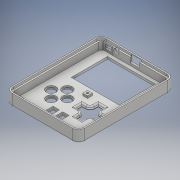
# Autodesk Inventor part: CaseGroboyFront
Saved by Autodesk Inventor 2017 SP1 (Build 210196100, 196)
## iProperties
Created: 2017-08-23
Part Number: CaseGroboyFront
Material: Generic
Document SubType Name: Modeling
Designer: Groguard
Density: 1 g/cm^3
Appearance: Default
Author: Groguard
Autodesk Inventor part; units mm, degrees
ref_plane "YZ Plane" through (0, 0, 0) normal (1, 0, 0) x (0, 1, 0)
ref_plane "XZ Plane" through (0, 0, 0) normal (0, 1, 0) x (-1, 0, 0)
ref_plane "XY Plane" through (0, 0, 0) normal (0, 0, 1) x (1, 0, 0)
sketch "Sketch1" plane through (0, 0, 0) normal (0, 0, 1) x (1, 0, 0)
  line L0 (50, 18.25) -> (50, 11.75)
  arc A0 (50.0508, 18.25) -> (49.9492, 18.25) centre (50, 18.25) ccw
  line L1 (50, 11.75) -> (44, 11.75)
  line L2 (44, 11.75) -> (44, 18.25)
  arc A1 (44.0508, 18.25) -> (43.9492, 18.25) centre (44, 18.25) ccw
  line L3 (44, 18.25) -> (50, 18.25)
  arc A2 (50, 18.1992) -> (50, 18.3008) centre (50, 18.25) ccw
  arc A3 (44, 18.3008) -> (44, 18.1992) centre (44, 18.25) ccw
  line L4 (38, 18.25) -> (38, 11.75)
  arc A4 (38.0508, 18.25) -> (37.9492, 18.25) centre (38, 18.25) ccw
  line L5 (38, 11.75) -> (32, 11.75)
  line L6 (32, 11.75) -> (32, 18.25)
  arc A5 (32.0508, 18.25) -> (31.9492, 18.25) centre (32, 18.25) ccw
  line L7 (32, 18.25) -> (38, 18.25)
  arc A6 (38, 18.1992) -> (38, 18.3008) centre (38, 18.25) ccw
  arc A7 (32, 18.3008) -> (32, 18.1992) centre (32, 18.25) ccw
  line L8 (3.96, 108.28) -> (73.16, 108.28)
  arc A8 (73.16, 108.2482) -> (73.16, 108.3118) centre (73.16, 108.28) ccw
  arc A9 (3.96, 108.3118) -> (3.96, 108.2482) centre (3.96, 108.28) ccw
  line L9 (73.16, 108.28) -> (73.16, 58.28)
  arc A10 (73.1282, 58.28) -> (73.1917, 58.28) centre (73.16, 58.28) ccw
  arc A11 (73.1917, 108.28) -> (73.1282, 108.28) centre (73.16, 108.28) ccw
  line L10 (73.16, 58.28) -> (3.96, 58.28)
  arc A12 (3.96, 58.3118) -> (3.96, 58.2482) centre (3.96, 58.28) ccw
  arc A13 (73.16, 58.2482) -> (73.16, 58.3118) centre (73.16, 58.28) ccw
  line L11 (3.96, 58.28) -> (3.96, 108.28)
  arc A14 (3.9918, 108.28) -> (3.9283, 108.28) centre (3.96, 108.28) ccw
  arc A15 (3.9283, 58.28) -> (3.9918, 58.28) centre (3.96, 58.28) ccw
  line L12 (32, 18.25) -> (38, 18.25)
  line L13 (38, 18.25) -> (38, 11.75)
  line L14 (38, 11.75) -> (32, 11.75)
  line L15 (32, 11.75) -> (32, 18.25)
  line L16 (44, 18.25) -> (50, 18.25)
  line L17 (50, 18.25) -> (50, 11.75)
  line L18 (50, 11.75) -> (44, 11.75)
  line L19 (44, 11.75) -> (44, 18.25)
  arc A16 (83, 106.5858) -> (78.5858, 111) centre (78.5858, 106.5858) ccw
  line L20 (83, 106.5858) -> (83, 3.4142)
  arc A17 (78.5858, -1) -> (83, 3.4142) centre (78.5858, 3.4142) ccw
  line L21 (78.5858, -1) -> (3.4142, -1)
  arc A18 (-1, 3.4142) -> (3.4142, -1) centre (3.4142, 3.4142) ccw
  line L22 (-1, 3.4142) -> (-1, 106.5858)
  arc A19 (3.4142, 111) -> (-1, 106.5858) centre (3.4142, 106.5858) ccw
  line L23 (3.4142, 111) -> (78.5858, 111)
  arc A20 (86, 106.5858) -> (78.5858, 114) centre (78.5858, 106.5858) ccw
  line L24 (86, 106.5858) -> (86, 3.4142)
  arc A21 (78.5858, -4) -> (86, 3.4142) centre (78.5858, 3.4142) ccw
  line L25 (78.5858, -4) -> (3.4142, -4)
  arc A22 (-4, 3.4142) -> (3.4142, -4) centre (3.4142, 3.4142) ccw
  line L26 (-4, 3.4142) -> (-4, 106.5858)
  arc A23 (3.4142, 114) -> (-4, 106.5858) centre (3.4142, 106.5858) ccw
  line L27 (3.4142, 114) -> (78.5858, 114)
  line L28 (50.75, 39.3006) -> (46.75, 39.3006)
  line L29 (46.75, 39.3006) -> (46.75, 32.8006)
  line L30 (46.75, 32.8006) -> (50.75, 32.8006)
  line L31 (56.75, 26.8006) -> (56.75, 22.8006)
  line L32 (56.75, 45.3006) -> (56.75, 49.3006)
  line L33 (56.75, 49.3006) -> (63.25, 49.3006)
  line L34 (63.25, 49.3006) -> (63.25, 45.3006)
  line L35 (69.25, 39.3006) -> (73.25, 39.3006)
  line L36 (73.25, 39.3006) -> (73.25, 32.8006)
  line L37 (73.25, 32.8006) -> (69.25, 32.8006)
  line L38 (63.25, 26.8006) -> (63.25, 22.8006)
  line L39 (63.25, 22.8006) -> (56.75, 22.8006)
  arc A24 (63.25, 45.3006) -> (69.25, 39.3006) centre (69.25, 45.3006) ccw
  arc A25 (50.75, 39.3006) -> (56.75, 45.3006) centre (50.75, 45.3006) ccw
  arc A26 (56.75, 26.8006) -> (50.75, 32.8006) centre (50.75, 26.8006) ccw
  arc A27 (69.25, 32.8006) -> (63.25, 26.8006) centre (69.25, 26.8006) ccw
  circle A28 centre (22, 46) radius 5
  circle A29 centre (32, 36) radius 5
  circle A30 centre (22, 26) radius 5
  circle A31 centre (12, 36) radius 5
  line L40 (11.35, 60.9) -> (11.35, 105.9)
  line L41 (11.35, 105.9) -> (70.65, 105.9)
  line L42 (70.65, 105.9) -> (70.65, 60.9)
  line L43 (70.65, 60.9) -> (11.35, 60.9)
  point P0 (0, 0)
  point P1 (18.75, 39)
  point P2 (18.75, 32.5)
  point P3 (63.25, 39)
  point P4 (63.25, 32.5)
  constraints: 88 end point, 56 point on circle, 32 centre point, 4 parallel, 3 perpendicular, 2 horizontal, 1 point on line
extrude "Face" add sketch "Sketch1" along normal blind 3 contours L3 A0 A2 L0 | L3 L2 A3 A1 | L7 A4 A6 L4 | L7 L6 A7 A5 | L11 A9 A14 L8 | L8 L9 L10 L11 | A11 A8 L9 L8 | L11 L10 A15 A12 | A13 A10 L10 L9 | L20 A17 L21 A18 L22 A19 L23 A16 | L24 A21 L25 A22 L26 A23 L27 A20 | L40 L41 L42 L43
sketch "Sketch12" plane through (0, 0, 3) normal (0, 0, 1) x (1, 0, 0)
  line L0 (78.5858, 114) -> (3.4142, 114) projected
  line L1 (3.4142, 114) -> (78.5858, 114)
  arc A0 (86, 106.5858) -> (78.5858, 114) centre (78.5858, 106.5858) ccw projected
  arc A1 (86, 106.5858) -> (78.5858, 114) centre (78.5858, 106.5858) ccw
  line L2 (86, 3.4142) -> (86, 106.5858) projected
  line L3 (86, 106.5858) -> (86, 3.4142)
  arc A2 (78.5858, -4) -> (78.5858, -4) centre (78.5858, 3.4142) ccw
  line L4 (78.5858, -4) -> (3.4142, -4) projected
  line L5 (3.4142, -4) -> (78.5858, -4) projected
  line L6 (78.5858, -4) -> (3.4142, -4)
  arc A3 (-4, 3.4142) -> (3.4142, -4) centre (3.4142, 3.4142) ccw projected
  arc A4 (-4, 3.4142) -> (3.4142, -4) centre (3.4142, 3.4142) ccw
  line L7 (-4, 3.4142) -> (-4, 106.5858)
  line L8 (-4, 3.4142) -> (-4, 106.5858) projected
  arc A5 (3.4142, 114) -> (-4, 106.5858) centre (3.4142, 106.5858) ccw
  arc A6 (78.5858, -4) -> (86, 3.4142) centre (78.5858, 3.4142) ccw
  line L9 (-1, 106.5858) -> (-1, 3.4142)
  arc A7 (-1, 3.4142) -> (3.4142, -1) centre (3.4142, 3.4142) ccw
  line L10 (3.4142, -1) -> (78.5858, -1)
  arc A8 (78.5858, -1) -> (83, 3.4142) centre (78.5858, 3.4142) ccw
  line L11 (83, 3.4142) -> (83, 106.5858)
  arc A9 (83, 106.5858) -> (78.5858, 111) centre (78.5858, 106.5858) ccw
  line L12 (78.5858, 111) -> (3.4142, 111)
  arc A10 (3.4142, 111) -> (-1, 106.5858) centre (3.4142, 106.5858) ccw
  point P0 (0, 0)
  dimension "d70" = 3
  constraints: 16 end point, 16 point on circle, 8 centre point, 3 collinear, 1 vertical, 1 vertical alignment, 10 other
  measures "d70" radial gap between concentric circles of A5 A10
extrude "Walls" add sketch "Sketch12" along normal blind 12 contours A0 L2 A2 L11 A9 L12 A10 L9 A7 L10 L4 A3 L7 A5 L0 | A2 L10 A8 L11 picked at (75.0084, -1.4191)
sketch "Sketch14" plane through (0, 0, 15) normal (0, 0, 1) x (1, 0, 0)
  line L0 (78.5858, 114) -> (3.4142, 114)
  arc A0 (86, 106.5858) -> (78.5858, 114) centre (78.5858, 106.5858) ccw
  line L1 (86, 3.4142) -> (86, 106.5858)
  line L2 (3.4142, -4) -> (78.5858, -4)
  arc A1 (-4, 3.4142) -> (3.4142, -4) centre (3.4142, 3.4142) ccw
  line L3 (-4, 3.4142) -> (-4, 106.5858)
  arc A2 (3.4142, 114) -> (-4, 106.5858) centre (3.4142, 106.5858) ccw
  arc A3 (78.5858, -4) -> (86, 3.4142) centre (78.5858, 3.4142) ccw
  line L4 (-2.5, 106.5858) -> (-2.5, 3.4142)
  arc A4 (-2.5, 3.4142) -> (3.4142, -2.5) centre (3.4142, 3.4142) ccw
  line L5 (3.4142, -2.5) -> (78.5858, -2.5)
  arc A5 (78.5858, -2.5) -> (84.5, 3.4142) centre (78.5858, 3.4142) ccw
  line L6 (84.5, 3.4142) -> (84.5, 106.5858)
  arc A6 (84.5, 106.5858) -> (78.5858, 112.5) centre (78.5858, 106.5858) ccw
  line L7 (78.5858, 112.5) -> (3.4142, 112.5)
  arc A7 (3.4142, 112.5) -> (-2.5, 106.5858) centre (3.4142, 106.5858) ccw
  line L8 (-1, 106.5858) -> (-1, 3.4142)
  arc A8 (-1, 3.4142) -> (3.4142, -1) centre (3.4142, 3.4142) ccw
  line L9 (3.4142, -1) -> (78.5858, -1)
  arc A9 (78.5858, -1) -> (83, 3.4142) centre (78.5858, 3.4142) ccw
  line L10 (83, 3.4142) -> (83, 106.5858)
  arc A10 (83, 106.5858) -> (78.5858, 111) centre (78.5858, 106.5858) ccw
  line L11 (78.5858, 111) -> (3.4142, 111)
  arc A11 (3.4142, 111) -> (-1, 106.5858) centre (3.4142, 106.5858) ccw
  point P0 (0, 0)
  dimension "d73" = 1.5
  dimension "d74" = 3
  constraints: 24 end point, 24 point on circle, 12 centre point, 1 vertical, 14 other
  measures "d73" radial gap between concentric circles of A2 A7
  measures "d74" radial gap between concentric circles of A2 A11
extrude "Wall Lip" cut sketch "Sketch14" against normal blind 3 contours A7 L7 A6 L6 A5 L5 A4 L4
sketch "Sketch15" plane through (3.4142, 111, 3) normal (0, -1, 0) x (1, 0, 0)
  line L0 (0, 2) -> (8, 2)
  line L1 (8, 2) -> (8, 7)
  line L2 (8, 7) -> (0, 7)
  line L3 (0, 7) -> (0, 2)
  circle A0 centre (14.75, 6.5) radius 3.25
  line L4 (37.5858, 0) -> (37.5858, 5)
  line L5 (37.5827, 3) -> (31.5827, 3)
  line L6 (31.5827, 3) -> (43.5827, 3)
  line L7 (43.5827, 3) -> (43.5827, 11)
  line L8 (43.5827, 11) -> (31.5827, 11)
  line L9 (31.5827, 11) -> (31.5827, 3)
  line L10 (0.0031, 4) -> (0, 2)
  line L11 (75.1716, 0) -> (0, 0) projected
  line L12 (14.75, 0) -> (14.75, 6.5)
  line L13 (14.75, 0) -> (21.25, 0) construction
  point P0 (-3.4142, -3)
  dimension "d79" = 8
  dimension "d80" = 5
  dimension "d86" = 6.5
  dimension "d87" = 5
  dimension "d88" = 6
  dimension "d89" = 12
  dimension "d90" = 8
  dimension "d129" = 2
  dimension "d158" = 6.5
  dimension "d159" = 90
  constraints: 26 end point, 4 horizontal, 4 parallel, 4 perpendicular, 1 centre point, 1 point on line, 1 vertical
  measures "d79" distance of L2.end L1.end
  measures "d80" distance of L1.end L0.end
  measures "d86" diameter of A0
  measures "d87" distance of L4.end L4.start
  measures "d88" distance of L5.start L5.end
  measures "d89" distance of L8.end L7.end
  measures "d90" distance of L7.end L6.end
  measures "d129" distance of L10.start L10.end
  measures "d158" distance of L12.start L12.end
  measures "d159" angle of L13 L12
extrude "Power/Headphone" cut sketch "Sketch15" against normal blind 3
sketch "Sketch16" plane through (0, 0, 3) normal (0, 0, 1) x (1, 0, 0)
  line L0 (50, 11.75) -> (44, 11.75)
  circle A0 centre (22, 46) radius 6
  circle A1 centre (12, 36) radius 6
  circle A2 centre (22, 26) radius 6
  circle A3 centre (32, 36) radius 6
  line L1 (45.75, 40.3006) -> (50.75, 40.3006)
  arc A4 (50.75, 40.3006) -> (55.75, 45.3006) centre (50.75, 45.3006) ccw
  line L2 (55.75, 45.3006) -> (55.75, 50.3006)
  line L3 (55.75, 50.3006) -> (64.25, 50.3006)
  line L4 (64.25, 50.3006) -> (64.25, 45.3006)
  arc A5 (64.25, 45.3006) -> (69.25, 40.3006) centre (69.25, 45.3006) ccw
  line L5 (69.25, 40.3006) -> (74.25, 40.3006)
  line L6 (74.25, 40.3006) -> (74.25, 31.8006)
  line L7 (74.25, 31.8006) -> (69.25, 31.8006)
  arc A6 (69.25, 31.8006) -> (64.25, 26.8006) centre (69.25, 26.8006) ccw
  line L8 (64.25, 26.8006) -> (64.25, 21.8006)
  line L9 (64.25, 21.8006) -> (55.75, 21.8006)
  line L10 (55.75, 21.8006) -> (55.75, 26.8006)
  arc A7 (55.75, 26.8006) -> (50.75, 31.8006) centre (50.75, 26.8006) ccw
  line L11 (50.75, 31.8006) -> (45.75, 31.8006)
  line L12 (45.75, 31.8006) -> (45.75, 40.3006)
  line L13 (31, 10.75) -> (31, 19.25)
  line L14 (31, 19.25) -> (39, 19.25)
  line L15 (39, 19.25) -> (39, 10.75)
  line L16 (39, 10.75) -> (31, 10.75)
  line L17 (43, 10.75) -> (43, 19.25)
  line L18 (43, 19.25) -> (51, 19.25)
  line L19 (51, 19.25) -> (51, 10.75)
  line L20 (51, 10.75) -> (43, 10.75)
  line L21 (46.75, 39.3006) -> (50.75, 39.3006)
  arc A8 (50.75, 39.3006) -> (56.75, 45.3006) centre (50.75, 45.3006) ccw
  line L22 (56.75, 45.3006) -> (56.75, 49.3006)
  line L23 (56.75, 49.3006) -> (63.25, 49.3006)
  line L24 (63.25, 49.3006) -> (63.25, 45.3006)
  arc A9 (63.25, 45.3006) -> (69.25, 39.3006) centre (69.25, 45.3006) ccw
  line L25 (69.25, 39.3006) -> (73.25, 39.3006)
  line L26 (73.25, 39.3006) -> (73.25, 32.8006)
  line L27 (73.25, 32.8006) -> (69.25, 32.8006)
  arc A10 (69.25, 32.8006) -> (63.25, 26.8006) centre (69.25, 26.8006) ccw
  line L28 (63.25, 26.8006) -> (63.25, 22.8006)
  line L29 (63.25, 22.8006) -> (56.75, 22.8006)
  line L30 (56.75, 22.8006) -> (56.75, 26.8006)
  arc A11 (56.75, 26.8006) -> (50.75, 32.8006) centre (50.75, 26.8006) ccw
  line L31 (50.75, 32.8006) -> (46.75, 32.8006)
  line L32 (46.75, 32.8006) -> (46.75, 39.3006)
  circle A12 centre (22, 46) radius 5
  circle A13 centre (12, 36) radius 5
  circle A14 centre (22, 26) radius 5
  circle A15 centre (32, 36) radius 5
  line L33 (38, 18.25) -> (32, 18.25)
  line L34 (32, 18.25) -> (32, 11.75)
  line L35 (32, 11.75) -> (38, 11.75)
  line L36 (38, 11.75) -> (38, 18.25)
  line L37 (50, 18.25) -> (44, 18.25)
  line L38 (44, 18.25) -> (44, 11.75)
  line L39 (44, 11.75) -> (50, 11.75)
  line L40 (50, 11.75) -> (50, 18.25)
  point P0 (0, 0)
  point P1 (18.75, 39)
  point P2 (18.75, 32.5)
  point P3 (63.25, 39)
  point P4 (63.25, 32.5)
  dimension "d100" = 1
  dimension "d101" = 1
  dimension "d102" = 1
  dimension "d103" = 1
  dimension "d104" = 1
  dimension "d105" = 1
  dimension "d106" = 1
  constraints: 82 end point, 16 centre point, 16 point on circle, 8 parallel, 4 perpendicular, 21 other
  measures "d100" distance between parallel lines of L12 L32
  measures "d101" radial gap between concentric circles of A0 A12
  measures "d102" radial gap between concentric circles of A1 A13
  measures "d103" radial gap between concentric circles of A2 A14
  measures "d104" radial gap between concentric circles of A3 A15
  measures "d105" distance between parallel lines of L14 L33
  measures "d106" distance between parallel lines of L18 L37
extrude "Extrusion16" cut sketch "Sketch16" against normal blind 1.5
fillet "Fillet3" radius 2 8 edges at (-1.8284, 111.8284, 0) (41, 114, 0) (83.8284, 111.8284, 0) (86, 55, 0) (83.8284, -1.8284, 0) (41, -4, 0) (-1.8284, -1.8284, 0) (-4, 55, 0)
sketch "Sketch17" plane through (0, 0, 3) normal (0, 0, 1) x (1, 0, 0)
  line L0 (3.4142, -1) -> (78.5858, -1) projected
  line L1 (38, 49) -> (44, 49)
  line L2 (44, 49) -> (44, 55)
  line L3 (44, 55) -> (38, 55)
  line L4 (38, 55) -> (38, 49)
  line L5 (38, 49) -> (44, 55) construction
  line L6 (44, 49) -> (38, 55) construction
  line L7 (1, 1) -> (7, 1)
  line L8 (7, 1) -> (7, 7)
  line L9 (7, 7) -> (1, 7)
  line L10 (1, 7) -> (1, 1)
  line L11 (1, 1) -> (7, 7) construction
  line L12 (7, 1) -> (1, 7) construction
  line L13 (75, 1) -> (81, 1)
  line L14 (81, 1) -> (81, 7)
  line L15 (81, 7) -> (75, 7)
  line L16 (75, 7) -> (75, 1)
  line L17 (75, 1) -> (81, 7) construction
  line L18 (81, 1) -> (75, 7) construction
  circle A0 centre (41, 52) radius 1.375
  circle A1 centre (4, 4) radius 1.375
  circle A2 centre (78, 4) radius 1.375
  point P0 (0, 0)
  dimension "d115" = 6
  dimension "d116" = 6
  dimension "d117" = 6
  dimension "d118" = 6
  dimension "d119" = 6
  dimension "d120" = 6
  dimension "d121" = 2.75
  dimension "d122" = 2.75
  dimension "d123" = 2.75
  constraints: 36 end point, 6 parallel, 3 centre point, 3 horizontal, 3 perpendicular
  measures "d115" distance of L3.end L2.end
  measures "d116" distance of L2.end L1.end
  measures "d117" distance of L9.end L8.end
  measures "d118" distance of L8.end L7.end
  measures "d119" distance of L15.end L14.end
  measures "d120" distance of L14.end L13.end
  measures "d121" diameter of A0
  measures "d122" diameter of A1
  measures "d123" diameter of A2
extrude "Extrusion17" add sketch "Sketch17" along normal blind 2.7
sketch "Sketch18" plane through (0, 0, 3) normal (0, 0, 1) x (1, 0, 0)
  line L0 (-1, 106.5858) -> (-1, 3.4142)
  arc A0 (-1, 3.4142) -> (3.4142, -1) centre (3.4142, 3.4142) ccw
  line L1 (3.4142, -1) -> (78.5858, -1)
  arc A1 (78.5858, -1) -> (83, 3.4142) centre (78.5858, 3.4142) ccw
  line L2 (83, 3.4142) -> (83, 106.5858)
  arc A2 (83, 106.5858) -> (78.5858, 111) centre (78.5858, 106.5858) ccw
  line L3 (78.5858, 111) -> (3.4142, 111)
  arc A3 (3.4142, 111) -> (-1, 106.5858) centre (3.4142, 106.5858) ccw
  line L4 (-0.6, 3.4142) -> (-0.6, 106.5858)
  arc A4 (3.4142, 110.6) -> (-0.6, 106.5858) centre (3.4142, 106.5858) ccw
  line L5 (3.4142, 110.6) -> (78.5858, 110.6)
  arc A5 (82.6, 106.5858) -> (78.5858, 110.6) centre (78.5858, 106.5858) ccw
  line L6 (82.6, 106.5858) -> (82.6, 3.4142)
  arc A6 (78.5858, -0.6) -> (82.6, 3.4142) centre (78.5858, 3.4142) ccw
  line L7 (78.5858, -0.6) -> (3.4142, -0.6)
  arc A7 (-0.6, 3.4142) -> (3.4142, -0.6) centre (3.4142, 3.4142) ccw
  point P0 (0, 0)
  dimension "d126" = 0.4
  constraints: 16 end point, 16 point on circle, 8 centre point, 7 other
  measures "d126" distance between parallel lines of L0 L4
extrude "Extrusion18" add sketch "Sketch18" along normal blind 9
sketch "Sketch19" plane through (18.1642, 111, 9.5) normal (0, 1, 0) x (-1, 0, 0)
  circle A0 centre (0, 0) radius 3.25
  line L0 (14.75, 0.5) -> (6.75, 0.5) projected
  line L1 (14.75, -6.5) -> (14.75, 2.5) projected
  line L2 (6.75, -4.4993) -> (14.75, -4.4993)
  line L3 (14.75, -4.4993) -> (14.75, 0.5007)
  line L4 (14.75, 0.5007) -> (6.75, 0.5007)
  line L5 (6.75, 0.5007) -> (6.75, -4.4993)
  line L6 (-28.8327, 4.5) -> (-28.8327, 2.5) projected
  line L7 (-28.8327, -3.5) -> (-16.8327, -3.5) projected
  line L8 (-28.8327, 4.5) -> (-16.8327, 4.5)
  line L9 (-16.8327, 4.5) -> (-16.8327, -3.5)
  line L10 (-16.8327, -3.5) -> (-28.8327, -3.5)
  line L11 (-28.8327, -3.5) -> (-28.8327, 4.5)
  point P0 (18.1642, -9.5)
  dimension "d130" = 5
  constraints: 16 end point, 4 parallel, 2 horizontal, 2 perpendicular, 1 centre point
  measures "d130" distance of L2.end L3.end
extrude "Extrusion19" cut sketch "Sketch19" against normal blind 2
fillet "Fillet6" radius 1 4 edges at (46.9969, 114, 10) (40.9969, 114, 14) (34.9969, 114, 10) (40.9969, 114, 6)
fillet "Fillet7" radius 1 1 edges at (14.9142, 114, 9.5)
sketch "Sketch20" plane through (3.4142, 110.6, 3) normal (0, -1, 0) x (1, 0, 0)
  line L0 (0, 2.01) -> (8, 2.01)
  line L1 (8, 2.01) -> (8, 7)
  line L2 (8, 7) -> (0, 7)
  line L3 (0, 7) -> (0, 2.01)
  line L4 (0.0031, 4) -> (0, 2)
  line L5 (-2, 9) -> (10, 9)
  line L6 (10, 9) -> (10, 0.01)
  line L7 (10, 0.01) -> (-2, 0.01)
  line L8 (-2, 0.01) -> (-2, 9)
  point P0 (-3.4142, -3)
  dimension "d138" = 8
  dimension "d139" = 4.99
  dimension "d140" = 2
  dimension "d141" = 2
  constraints: 18 end point, 4 parallel, 2 perpendicular, 1 horizontal, 3 other
  measures "d138" distance of L2.end L1.end
  measures "d139" distance of L1.end L1.start
  measures "d140" distance of L4.start L4.end
  measures "d141" distance between parallel lines of L2 L5
extrude "Extrusion20" cut sketch "Sketch20" along normal mid plane 1.5
sketch "Sketch21" plane through (41, 52, 3) normal (0, 0, 1) x (1, 0, 0)
  circle A0 centre (-37, -48) radius 1.375 projected
  circle A1 centre (-37, -48) radius 1.375
  circle A2 centre (37, -48) radius 1.375 projected
  circle A3 centre (37, -48) radius 1.375
  circle A4 centre (0, 0) radius 1.375 projected
  circle A5 centre (0, 0) radius 1.375
  point P0 (-41, -52)
  constraints: 3 centre point, 3 coincident
extrude "Extrusion21" cut sketch "Sketch21" against normal blind 1.5
fillet "Fillet8" radius 2 16 edges at (45.75, 36.0506, 3) (48.25, 40.3006, 3) (54.2855, 41.7651, 3) (55.75, 47.8006, 3) (60, 50.3006, 3) (64.25, 47.8006, 3) (65.7145, 41.7651, 3) (71.75, 40.3006, 3) (74.25, 36.0506, 3) (71.75, 31.8006, 3) (65.7145, 30.3361, 3) (64.25, 24.3006, 3) (60, 21.8006, 3) (55.75, 24.3006, 3) (54.2855, 30.3361, 3) (48.25, 31.8006, 3)
fillet "Fillet9" radius 1 16 edges at (46.75, 36.0506, 1.5) (48.75, 39.3006, 1.5) (54.9926, 41.058, 1.5) (56.75, 47.3006, 1.5) (60, 49.3006, 1.5) (63.25, 47.3006, 1.5) (65.0074, 41.058, 1.5) (71.25, 39.3006, 1.5) (73.25, 36.0506, 1.5) (71.25, 32.8006, 1.5) (65.0074, 31.0432, 1.5) (63.25, 24.8006, 1.5) (60, 22.8006, 1.5) (56.75, 24.8006, 1.5) (54.9926, 31.0432, 1.5) (48.75, 32.8006, 1.5)
sketch "Sketch22" plane through (0, 0, 3) normal (0, 0, 1) x (1, 0, 0)
  line L0 (3.96, 108.28) -> (73.16, 108.28)
  arc A0 (73.16, 108.2482) -> (73.16, 108.3118) centre (73.16, 108.28) ccw
  arc A1 (3.96, 108.3118) -> (3.96, 108.2482) centre (3.96, 108.28) ccw
  line L1 (73.16, 108.28) -> (73.16, 58.28)
  arc A2 (73.1282, 58.28) -> (73.1917, 58.28) centre (73.16, 58.28) ccw
  arc A3 (73.1917, 108.28) -> (73.1282, 108.28) centre (73.16, 108.28) ccw
  line L2 (73.16, 58.28) -> (3.96, 58.28)
  arc A4 (3.96, 58.3118) -> (3.96, 58.2482) centre (3.96, 58.28) ccw
  arc A5 (73.16, 58.2482) -> (73.16, 58.3118) centre (73.16, 58.28) ccw
  line L3 (3.96, 58.28) -> (3.96, 108.28)
  arc A6 (3.9918, 108.28) -> (3.9283, 108.28) centre (3.96, 108.28) ccw
  arc A7 (3.9283, 58.28) -> (3.9918, 58.28) centre (3.96, 58.28) ccw
  line L4 (11.35, 61.4) -> (11.35, 106.4)
  line L5 (11.35, 106.4) -> (70.65, 106.4)
  line L6 (70.65, 106.4) -> (70.65, 61.4)
  line L7 (70.65, 61.4) -> (11.35, 61.4)
  point P0 (0, 0)
  point P1 (3.4142, 106.5858)
  constraints: 16 end point, 16 point on circle, 8 centre point, 1 perpendicular
extrude "Extrusion22" cut sketch "Sketch22" against normal blind 3 contours L4 L5 L6 L7
body "Solid3"
